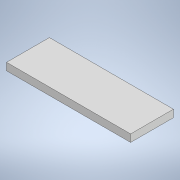
# Autodesk Inventor part: controllerBottom
Saved by Autodesk Inventor 2021 (Build 250183000, 183)
## iProperties
Created: 2024-03-20
Part Number: controllerBottom
Material: Generic
Document SubType Name: Modeling
Designer: 21seblin
Density: 1 g/cm^3
Appearance: Default
Author: 21seblin
Autodesk Inventor part; units mm, degrees
ref_plane "YZ Plane" through (0, 0, 0) normal (1, 0, 0) x (0, 1, 0)
ref_plane "XZ Plane" through (0, 0, 0) normal (0, 1, 0) x (-1, 0, 0)
ref_plane "XY Plane" through (0, 0, 0) normal (0, 0, 1) x (1, 0, 0)
sketch "Sketch1" plane through (0, 0, 0) normal (0, 1, 0) x (-1, 0, 0)
  line L0 (82, -27) -> (-82, -27)
  line L1 (-82, -27) -> (-82, 27)
  line L2 (-82, 27) -> (82, 27)
  line L3 (82, 27) -> (82, -27)
  line L4 (82, -27) -> (-82, 27) construction
  line L5 (-82, -27) -> (82, 27) construction
  line L6 (82, 27) -> (82, 28.5)
  line L7 (82, 28.5) -> (69.3, 28.5)
  line L8 (69.3, 28.5) -> (65.3, 28.5)
  line L9 (65.3, 28.5) -> (65.3, 27)
  line L10 (65.3, 27) -> (69.3, 27)
  line L11 (69.3, 27) -> (69.3, 28.5)
  line L12 (2, 27) -> (2, 28.5)
  line L13 (2, 28.5) -> (-2, 28.5)
  line L14 (-2, 28.5) -> (-2, 27)
  line L15 (-65.3, 27) -> (-65.3, 28.5)
  line L16 (-65.3, 28.5) -> (-69.3, 28.5)
  line L17 (-69.3, 28.5) -> (-69.3, 27)
  point P0 (0, 0)
  dimension "d0" = 164
  dimension "d1" = 54
  dimension "d3" = 4
  dimension "d4" = 1.5
  dimension "d7" = 67.3
  constraints: 36 end point, 4 parallel, 3 horizontal, 3 perpendicular, 2 midpoint, 1 collinear, 1 point on line, 1 vertical, 13 other
  measures "d0" distance of L0.start L0.end
  measures "d1" distance of L0.end L1.end
  measures "d3" distance of L7.end L8.end
  measures "d4" distance of L8.end L9.end
  measures "d7" distance of L10.end L12.start
ref_plane "Work Plane1" through (0, 9, 0) normal (0, 1, 0) x (1, 0, 0)
sketch "Sketch2" plane through (0, 9, 0) normal (0, 1, 0) x (1, 0, 0)
  line L0 (-84, 29) -> (84, 29)
  line L1 (84, 29) -> (84, -29)
  line L2 (84, -29) -> (-84, -29)
  line L3 (-84, -29) -> (-84, 29)
  line L4 (-84, 29) -> (84, -29) construction
  line L5 (84, 29) -> (-84, -29) construction
  point P0 (0, 0)
  dimension "d14" = 168
  dimension "d15" = 58
  constraints: 12 end point, 2 midpoint, 2 parallel, 1 horizontal, 1 perpendicular
  measures "d14" distance of L0.start L0.end
  measures "d15" distance of L0.end L1.end
extrude "Extrusion2" add sketch "Sketch2" along normal blind 10
extrude "Extrusion3" cut sketch "Sketch1" along normal blind 18 contours L0 L1 L2 L3 | L2 L9 L8 L11 | L17 L16 L15 L2 | L2 L14 L13 L12
body "Solid1"
